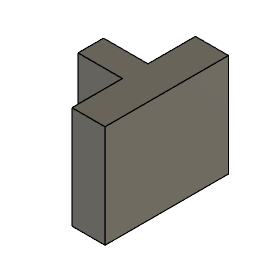
Assembly - JST version (Autodesk Fusion 360 archive; units mm, degrees)
design "Button"
Autodesk Fusion 360 part; units mm, degrees
sketch "Sketch1" plane through (0, 0, 0) normal (0, 0, 1) x (1, 0, 0)
  line L0 (-1.05, 4.05) -> (1.15, 4.05)
  line L1 (1.15, 4.05) -> (1.15, -4.15)
  line L2 (1.15, -4.15) -> (-1.05, -4.15)
  line L3 (-1.05, 0.9) -> (-4, 0.9)
  line L4 (-4, 0.9) -> (-4, -0.8)
  line L5 (-4, -0.8) -> (-1.05, -0.8)
  line L6 (1.15, -0.9) -> (1.15, 0.9)
  line L7 (-1.05, -4.15) -> (-1.05, -0.8)
  line L8 (-1.05, 0.9) -> (-1.05, 4.05)
  dimension "d1" = 2.2
  dimension "d2" = 8.2
  dimension "d4" = 4.15
  dimension "d5" = 1.15
  dimension "d6" = 1.7
  dimension "d7" = 0.9
  dimension "d12" = 4
  constraint horizontal L0
  constraint vertical L1
  constraint horizontal L2
  constraint vertical L7
  constraint horizontal L3
  constraint vertical L4
  constraint horizontal L5
  constraint vertical L6
  constraint coincident L1 L6.end
  constraint collinear L7 L8
  measures "d1" distance of L0.start L0.end
  measures "d2" distance of L0.end L1.end
  measures "d4" distance of origin L2
  measures "d5" distance of origin L1
  measures "d6" distance of L3.end L4.end
  measures "d7" distance of origin L3
  measures "d12" distance of origin L4
extrude "Extrude1" add sketch "Sketch1" along normal blind 6.814
equation "d1 = 2.5 mm - 0.3 mm"
equation "d2 = 8.60 mm - 0.4 mm"
equation "d4 = ( 8.3 / 2 ) * 1 mm"
equation "d5 = ( 2.3 / 2 ) * 1 mm"
equation "d6 = 2 mm - 0.3 mm"
equation "d7 = ( 1.8 / 2 ) * 1 mm"
equation "d10 = 6.964 mm - 0.15 mm"
equation "d12 = 4.3 mm - 0.3 mm"

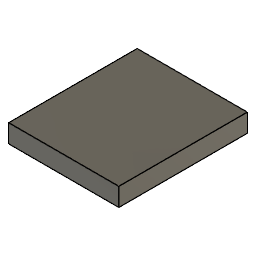
design "Battery"
Autodesk Fusion 360 part; units mm, degrees
sketch "Sketch1" plane through (0, 0, 0) normal (0, 0, 1) x (1, 0, 0)
  line L0 (0, 0) -> (30, 0)
  line L1 (30, 0) -> (30, -35)
  line L2 (30, -35) -> (0, -35)
  line L3 (0, -35) -> (0, 0)
  dimension "d1" = 35
  dimension "d2" = 30
  constraint horizontal L0
  constraint vertical L1
  constraint horizontal L2
  constraint vertical L3
  constraint coincident L0.start L3.end
  measures "d1" distance of L0.start L2.end
  measures "d2" distance of L0.start L0.end
extrude "Extrude1" add sketch "Sketch1" along normal blind 5

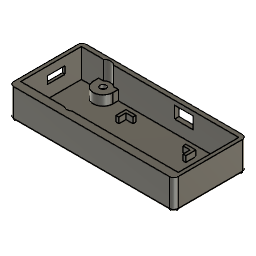
design "Base"
Autodesk Fusion 360 part; units mm, degrees
sketch "Sketch1" plane through (0, 0, 0) normal (0, 0, 1) x (1, 0, 0)
  line L0 (44.1755, -16.9975) -> (-44.1755, -16.9975)
  line L1 (-44.1755, -16.9975) -> (-44.1755, 16.9975)
  line L2 (-44.1755, 16.9975) -> (44.1755, 16.9975)
  line L3 (44.1755, 16.9975) -> (44.1755, -16.9975)
  line L4 (44.1755, -16.9975) -> (-44.1755, 16.9975) construction
  line L5 (-44.1755, -16.9975) -> (44.1755, 16.9975) construction
  line L6 (46.1755, -21.4975) -> (-46.1755, -21.4975)
  line L7 (-46.1755, -21.4975) -> (-46.1755, 19.4975)
  line L8 (-46.1755, 19.4975) -> (46.1755, 19.4975)
  line L9 (46.1755, 19.4975) -> (46.1755, -21.4975)
  dimension "d1" = 33.995
  dimension "d2" = 88.351
  constraint horizontal L0
  constraint perpendicular L0 L1
  constraint parallel L0 L2
  constraint parallel L1 L3
  constraint coincident L4 origin
  constraint coincident L5 origin
  measures "d1" distance of L0.end L1.end
  measures "d2" distance of L0.start L0.end
extrude "Extrude1" add sketch "Sketch1" against normal blind 1 contours L0 L1 L2 L3 | L6 L7 L8 L9
extrude "Extrude2" add sketch "Sketch1" along normal blind 16
sketch "Sketch2" plane through (0, 0, 0) normal (0, 0, 1) x (-1, 0, 0)
  line L0 (44.1755, -16.9975) -> (44.1755, 16.9975)
  line L1 (44.1755, 16.9975) -> (-44.1755, 16.9975)
  line L2 (-44.1755, 16.9975) -> (-44.1755, -16.9975)
  line L3 (-44.1755, -16.9975) -> (44.1755, -16.9975)
  circle A0 centre (28.9565, -13.9705) radius 1.7
  circle A1 centre (28.9565, -13.9705) radius 4
  circle A2 centre (28.9565, -13.9705) radius 5.5
  circle A3 centre (17.6535, 13.4625) radius 1.7
  circle A4 centre (17.6535, 13.4625) radius 4
  circle A5 centre (17.6535, 13.4625) radius 5.5
  circle A6 centre (-39.8785, 11.5575) radius 1.7
  circle A7 centre (-39.8785, 11.5575) radius 4
  circle A8 centre (-39.8785, 11.5575) radius 5.5
  line L4 (-34.3785, 11.5575) -> (-34.3785, 16.9975)
  line L5 (-39.8785, 6.0575) -> (-44.1755, 6.0575)
  line L6 (23.4565, -13.9705) -> (23.4565, -16.9975)
  line L7 (23.1535, 13.4625) -> (23.1535, 16.9975)
  line L8 (12.1535, 13.4625) -> (12.1535, 18.5)
  line L9 (34.4565, -13.9705) -> (34.4565, -18)
  dimension "d8" = 3.4
  dimension "d9" = 15.219
  dimension "d10" = 3.027
  dimension "d11" = 2.3
  dimension "d12" = 1.5
  dimension "d22" = 3.4
  dimension "d23" = 26.522
  dimension "d24" = 3.535
  dimension "d25" = 2.3
  dimension "d26" = 1.5
  dimension "d27" = 3.4
  dimension "d28" = 4.297
  dimension "d29" = 5.44
  dimension "d30" = 2.3
  dimension "d31" = 1.5
  constraint coincident A8 L4.start
  constraint coincident L1 L4.end
  constraint tangent A8 L4
  constraint perpendicular L1 L4
  constraint coincident A8 L5.start
  constraint coincident L2 L5.end
  constraint tangent A8 L5
  constraint perpendicular L2 L5
  constraint coincident A2 L6.start
  constraint coincident L3 L6.end
  constraint tangent A2 L6
  constraint perpendicular L3 L6
  constraint coincident A5 L7.start
  constraint coincident L1 L7.end
  constraint tangent A5 L7
  constraint perpendicular L1 L7
  constraint coincident A5 L8.start
  constraint tangent A5 L8
  constraint perpendicular L1 L8
  constraint coincident A2 L9.start
  constraint tangent A2 L9
  constraint perpendicular L3 L9
  measures "d8" diameter of A0
  measures "d9" distance of L0 A0.centre
  measures "d10" distance of L3 A0.centre
  measures "d22" diameter of A3
  measures "d23" distance of L0 A3.centre
  measures "d24" distance of L1 A3.centre
  measures "d27" diameter of A6
  measures "d28" distance of L2 A6.centre
  measures "d29" distance of L1 A6.centre
extrude "Extrude3" add sketch "Sketch2" along normal blind 5.5 contours L3 A2 L9 | L1 A5 L7 | L3 A1 A2 | L1 A4 A5 | L3 A2 L6 | L1 A5 L8 | L1 A8 L4 | L2 A8 L5 | L1 L2 A8 | L1 L2 A8 picked at (23.9776, -13.6565) picked at (13.0083, 11.6405)
extrude "Extrude4" cut sketch "Sketch2" along normal blind 5.5 contours L3 A1 | L3 A1 | L1 A4 | L1 A4 | A7
extrude "Extrude5" add sketch "Sketch2" along normal blind 2 from surface at 3.5 contours L3 A1 | L3 A1 | L1 A4 | L1 A4 | A7
extrude "Extrude6" cut sketch "Sketch2" against normal blind 9 contours L3 A1 | L3 A1 | L1 A4 | L1 A4 | A0 | A3 | A6 | A7
sketch "Sketch3" plane through (-46.1755, 0, 0) normal (-1, 0, 0) x (0, -1, 0)
  line L0 (-19.4975, 16) -> (-19.4975, -1)
  line L1 (-19.4975, -1) -> (21.4975, -1)
  line L2 (21.4975, -1) -> (21.4975, 16)
  line L3 (21.4975, 16) -> (-19.4975, 16)
  line L4 (-7.8915, 11.246) -> (2.0485, 11.246)
  line L5 (2.0485, 11.246) -> (2.0485, 7.086)
  line L6 (2.0485, 7.086) -> (-7.8915, 7.086)
  line L7 (-7.8915, 7.086) -> (-7.8915, 11.246)
  dimension "d32" = 9.94
  dimension "d33" = 4.16
  dimension "d36" = 11.606
  dimension "d42" = 8.086
  constraint horizontal L4
  constraint vertical L5
  constraint horizontal L6
  constraint vertical L7
  measures "d32" distance of L4.start L4.end
  measures "d33" distance of L4.start L6.end
  measures "d36" distance of L0 L7
  measures "d42" distance of L1 L6
extrude "Extrude7" cut sketch "Sketch3" against normal blind 6 contours L4 L5 L6 L7
chamfer "Chamfer1" distance 0.5 angle 45 4 edges at (-46.1755, 2.9215, 11.246) (-46.1755, -2.0485, 9.166) (-46.1755, 2.9215, 7.086) (-46.1755, 7.8915, 9.166) tangent chain off
sketch "Sketch5" plane through (0, 16.9975, 0) normal (0, -1, 0) x (1, 0, 0)
  line L0 (-34.4565, 5.5) -> (-23.4565, 5.5)
  line L1 (-23.4565, 5.5) -> (-23.4565, 0)
  line L2 (-23.4565, 0) -> (44.1755, 0)
  line L3 (44.1755, 0) -> (44.1755, 16)
  line L4 (44.1755, 16) -> (-44.1755, 16)
  line L5 (-44.1755, 16) -> (-44.1755, 0)
  line L6 (-44.1755, 0) -> (-34.4565, 0)
  line L7 (-34.4565, 0) -> (-34.4565, 5.5)
sketch "Sketch6" plane through (0, -16.9975, 0) normal (0, 1, 0) x (-1, 0, 0)
  line L0 (12.1535, 5.5) -> (23.1535, 5.5)
  line L1 (23.1535, 5.5) -> (23.1535, 0)
  line L2 (23.1535, 0) -> (44.1755, 0)
  line L3 (44.1755, 0) -> (44.1755, 16)
  line L4 (44.1755, 16) -> (-44.1755, 16)
  line L5 (-44.1755, 16) -> (-44.1755, 5.5)
  line L6 (-44.1755, 5.5) -> (-34.3785, 5.5)
  line L7 (-34.3785, 5.5) -> (-34.3785, 0)
  line L8 (-34.3785, 0) -> (12.1535, 0)
  line L9 (12.1535, 0) -> (12.1535, 5.5)
  line L10 (-34.3785, 5.5) -> (12.1535, 5.5)
  line L11 (12.1535, 5.5) -> (12.1535, 0)
  line L12 (12.1535, 0) -> (-34.3785, 0)
  line L13 (-34.3785, 0) -> (-34.3785, 5.5)
  constraint horizontal L10
  constraint vertical L11
  constraint horizontal L12
  constraint vertical L13
  constraint coincident L8.end L9.start
  constraint coincident L6.end L7.start
extrude "Extrude8" cut sketch "Sketch6" against normal blind 3.5 contours L7 L8 L9 L10 L11 L12 L13
chamfer "Chamfer2" distance 1.5 angle 45 1 edges at (11.1125, -16.9975, 5.5) tangent chain off
sketch "Sketch7" plane through (0, 0, 0) normal (0, 0, 1) x (-1, 0, 0)
  line L0 (34.4565, -13.9705) -> (34.4565, -16.9975)
  line L1 (34.4565, -16.9975) -> (44.1755, -16.9975)
  line L2 (44.1755, -16.9975) -> (44.1755, 16.9975)
  line L3 (44.1755, 16.9975) -> (23.1535, 16.9975)
  line L4 (23.1535, 16.9975) -> (23.1535, 13.4625)
  arc A0 (12.1535, 13.4625) -> (23.1535, 13.4625) centre (17.6535, 13.4625) ccw
  line L5 (12.1535, 13.4625) -> (12.1535, 20.4975)
  line L6 (12.1535, 20.4975) -> (-34.3785, 20.4975)
  line L7 (-34.3785, 20.4975) -> (-34.3785, 11.5575)
  arc A1 (-39.8785, 6.0575) -> (-34.3785, 11.5575) centre (-39.8785, 11.5575) ccw
  line L8 (-39.8785, 6.0575) -> (-44.1755, 6.0575)
  line L9 (-44.1755, 6.0575) -> (-44.1755, -16.9975)
  line L10 (23.4565, -16.9975) -> (23.4565, -13.9705)
  arc A2 (34.4565, -13.9705) -> (23.4565, -13.9705) centre (28.9565, -13.9705) ccw
  line L11 (-44.1755, 16.9975) -> (44.1755, 16.9975)
  line L12 (13.7535, -6.0025) -> (13.7535, -11.6025)
  line L13 (13.7535, -11.6025) -> (8.1535, -11.6025)
  line L14 (8.1535, -11.6025) -> (8.1535, -10.0025)
  line L15 (13.7535, -6.0025) -> (12.1535, -6.0025)
  line L16 (12.1535, -6.0025) -> (12.1535, -10.0025)
  line L17 (12.1535, -10.0025) -> (8.1535, -10.0025)
  line L18 (-19.8465, -11.6025) -> (-25.4465, -11.6025)
  line L19 (-25.4465, -11.6025) -> (-25.4465, -6.0025)
  line L20 (-25.4465, -6.0025) -> (-23.8465, -6.0025)
  line L21 (-19.8465, -11.6025) -> (-19.8465, -10.0025)
  line L22 (-23.8465, -6.0025) -> (-23.8465, -10.0025)
  line L23 (-23.8465, -10.0025) -> (-19.8465, -10.0025)
  line L24 (17, 20.4975) -> (-40, 20.4975)
  dimension "d69" = 5.6
  dimension "d70" = 5.6
  dimension "d71" = 1.6
  dimension "d72" = 1.6
  dimension "d73" = 1.6
  dimension "d74" = 5.6
  dimension "d75" = 5.6
  dimension "d76" = 1.6
  dimension "d77" = 1.6
  dimension "d82" = 36
  dimension "d84" = 3.5
  dimension "d85" = 30.5
  dimension "d86" = 30.5
  constraint perpendicular L6 L12
  constraint perpendicular L12 L13
  constraint perpendicular L13 L14
  constraint perpendicular L12 L15
  constraint perpendicular L15 L16
  constraint perpendicular L14 L17
  constraint horizontal L18
  constraint perpendicular L18 L19
  constraint perpendicular L19 L20
  constraint perpendicular L18 L21
  constraint perpendicular L20 L22
  constraint perpendicular L22 L23
  constraint perpendicular L4 L24
  measures "d69" distance of L12.start L12.end
  measures "d70" distance of L12.end L13.end
  measures "d71" distance of L13.end L14.end
  measures "d72" distance of L12.start L15.end
  measures "d73" distance of L5 L12
  measures "d74" distance of L18.start L18.end
  measures "d75" distance of L18.end L19.end
  measures "d76" distance of L18.start L21.end
  measures "d77" distance of L19.end L20.end
  measures "d82" distance of L16 L22
  measures "d84" distance of L11 L24
  measures "d85" distance of L17 L24
  measures "d86" distance of L23 L24
extrude "Extrude10" add sketch "Sketch7" along normal blind 3.25 contours L12 L13 L14 L15 L16 L17 | L18 L19 L20 L21 L22 L23
fillet "Fillet1" radius 2.5 4 edges at (46.1755, 19.4975, 7.5) (-46.1755, 19.4975, 7.5) (-46.1755, -21.4975, 7.5) (46.1755, -21.4975, 7.5)
fillet "Fillet2" radius 1.5 8 edges at (-45.4433, -20.7653, -1) (-46.1755, -1, -1) (-45.4433, 18.7653, -1) (0, 19.4975, -1) (45.4433, 18.7653, -1) (46.1755, -1, -1) (45.4433, -20.7653, -1) (0, -21.4975, -1)
sketch "Sketch9" plane through (0, 19.4975, 0) normal (0, 1, 0) x (-1, 0, 0)
  line L0 (-43.6755, 0.5) -> (43.6755, 0.5)
  line L1 (43.6755, 0.5) -> (43.6755, 16)
  line L2 (43.6755, 16) -> (-43.6755, 16)
  line L3 (-43.6755, 16) -> (-43.6755, 0.5)
  line L4 (-18.5144, 13.6041, 0.0269) -> (-8.1544, 13.6041, 0.0269)
  line L5 (-8.1544, 13.6041, 0.0269) -> (-8.1544, 6.9041, 0.0269)
  line L6 (-8.1544, 6.9041, 0.0269) -> (-18.5144, 6.9041, 0.0269)
  line L7 (-18.5144, 6.9041, 0.0269) -> (-18.5144, 13.6041, 0.0269)
  line L8 (-46.1754, 16.6041, 0.0269) -> (-46.1754, 0.6041, 0.0269)
  line L9 (-17.2989, 5.3181, 0.0269) -> (-9.2989, 5.3181, 0.0269)
  line L10 (-43.6755, -1, -1.5) -> (43.6755, -1, -1.5)
  line L11 (-45, -1.1818) -> (-2, -1.1818)
  dimension "d94" = 2.5
  dimension "d95" = 27.661
  dimension "d96" = 10.36
  dimension "d97" = 6.7
  dimension "d99" = 1.586
  dimension "d101" = 6.5
  constraint horizontal L11
extrude "Extrude11" cut sketch "Sketch9" against normal blind 6 contours L4 L5 L6 L7 in plane through (0, 19.5244, 0) normal (0, 1, 0)
sketch "Sketch10" plane through (0, 0, 5.5) normal (0, 0, 1) x (-1, 0, 0)
  circle A0 centre (28.9565, -13.9705) radius 1.7
  line L0 (23.4565, -13.9705) -> (23.4565, -16.9975)
  line L1 (23.4565, -16.9975) -> (34.4565, -16.9975)
  line L2 (34.4565, -16.9975) -> (34.4565, -13.9705)
  arc A1 (34.4565, -13.9705) -> (23.4565, -13.9705) centre (28.9565, -13.9705) ccw
  circle A2 centre (28.9565, -13.9705) radius 2.3
  circle A3 centre (28.9565, -13.9705) radius 3.9
  circle A4 centre (28.9565, -13.9705) radius 4.2
  circle A5 centre (-39.8785, 11.5575) radius 2.3
  arc A6 (-39.8785, 6.0575) -> (-34.3785, 11.5575) centre (-39.8785, 11.5575) ccw
  circle A7 centre (-39.8785, 11.5575) radius 3.9
  circle A8 centre (-39.8785, 11.5575) radius 4.2
  circle A9 centre (17.6535, 13.4625) radius 2.3
  circle A10 centre (17.6535, 13.4625) radius 1.7
  circle A11 centre (17.6535, 13.4625) radius 3.9
  circle A12 centre (17.6535, 13.4625) radius 4.2
  dimension "d102" = 4.6
  dimension "d103" = 1.6
  dimension "d104" = 0.3
  dimension "d105" = 4.6
  dimension "d106" = 1.6
  dimension "d107" = 0.3
  dimension "d108" = 4.6
  dimension "d110" = 1.6
  dimension "d111" = 0.3
  constraint concentric A0 A2
  constraint concentric A5 A6
  constraint coincident A9.centre A10.centre
  measures "d102" diameter of A2
  measures "d105" diameter of A5
  measures "d108" diameter of A9
extrude "Extrude12" cut sketch "Sketch10" along normal blind 17 contours L1 A3 A4 | L1 A3 A4 | L1 A3 | L1 A3 | A2 | A5 | A7 | A8 | A9 | A11 | A12
equation "d1 = 32.995 mm + 1 mm"
equation "d2 = 87.351 mm + 1 mm"
equation "d9 = 14.719 mm + 0.5 mm"
equation "d10 = 2.527 mm + 0.5 mm"
equation "d23 = 26.022 mm + 0.5 mm"
equation "d24 = 3.035 mm + 0.5 mm"
equation "d28 = 3.797 mm + 0.5 mm"
equation "d29 = 4.94 mm + 0.5 mm"
equation "d32 = 9.44 mm + 0.5 mm"
equation "d33 = 3.66 mm + 0.5 mm"
equation "d36 = 12.106 mm - 0.5 mm"
equation "d95 = 27.761 mm - 0.1 mm"
equation "d96 = 10.16 mm + 0.2 mm"
equation "d97 = 6.50 mm + 0.2 mm"
